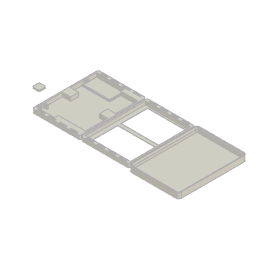
screensv16 (Autodesk Fusion 360 design; units mm, degrees)
Autodesk Fusion 360 part; units mm, degrees
sketch "Sketch1" plane through (0, 0, 0) normal (0, 0, 1) x (1, 0, 0)
  line L0 (0.0242, 17.1172) -> (73.5242, 17.1172)
  line L1 (73.5242, 17.1172) -> (73.5242, -31.8828)
  line L2 (73.5242, -31.8828) -> (0.0242, -31.8828)
  line L3 (0.0242, -31.8828) -> (0.0242, 17.1172)
  line L4 (-7.2758, 20.2172) -> (70.6242, 20.2172)
  line L5 (-7.2758, 20.2172) -> (75.7242, 20.2172)
  line L6 (75.7242, 20.2172) -> (75.7242, -34.9828)
  line L7 (-7.2758, -34.9828) -> (-7.2758, 20.2172)
  line L8 (-9.6758, 25.8172) -> (78.1242, 25.8172)
  line L9 (78.1242, 25.8172) -> (78.1242, -95.7828)
  line L10 (78.1242, -95.7828) -> (-9.6758, -95.7828)
  line L11 (-9.6758, -95.7828) -> (-9.6758, 25.8172)
  line L12 (-7.2758, -34.9828) -> (70.6242, -34.9828)
  line L13 (70.6242, -34.9828) -> (75.7242, -34.9828)
  line L14 (75.7242, -34.9828) -> (75.7242, -90.1828)
  line L15 (-7.2758, -90.1828) -> (70.6242, -90.1828)
  line L16 (70.6242, -90.1828) -> (75.7242, -90.1828)
  line L17 (-7.2758, -34.9828) -> (-7.2758, -90.1828)
  line L18 (0.0242, -38.0828) -> (73.5242, -38.0828)
  line L19 (73.5242, -38.0828) -> (73.5242, -87.0828)
  line L20 (73.5242, -87.0828) -> (0.0242, -87.0828)
  line L21 (0.0242, -87.0828) -> (0.0242, -38.0828)
  line L22 (70.9642, 22.0172) -> (57.9642, 22.0172)
  line L23 (57.9642, 22.0172) -> (57.9642, 24.0172)
  line L24 (57.9642, 24.0172) -> (70.9642, 24.0172)
  line L25 (70.9642, 24.0172) -> (70.9642, 22.0172)
  line L26 (10.4842, 22.0172) -> (-2.5158, 22.0172)
  line L27 (-2.5158, 22.0172) -> (-2.5158, 24.0172)
  line L28 (-2.5158, 24.0172) -> (10.4842, 24.0172)
  line L29 (10.4842, 24.0172) -> (10.4842, 22.0172)
  line L30 (50.8042, 22.0172) -> (37.8042, 22.0172)
  line L31 (37.8042, 22.0172) -> (37.8042, 24.0172)
  line L32 (37.8042, 24.0172) -> (50.8042, 24.0172)
  line L33 (50.8042, 24.0172) -> (50.8042, 22.0172)
  line L34 (30.6442, 22.0172) -> (17.6442, 22.0172)
  line L35 (17.6442, 22.0172) -> (17.6442, 24.0172)
  line L36 (17.6442, 24.0172) -> (30.6442, 24.0172)
  line L37 (30.6442, 24.0172) -> (30.6442, 22.0172)
  line L38 (70.9642, -93.9828) -> (57.9642, -93.9828)
  line L39 (57.9642, -93.9828) -> (57.9642, -91.9828)
  line L40 (57.9642, -91.9828) -> (70.9642, -91.9828)
  line L41 (70.9642, -91.9828) -> (70.9642, -93.9828)
  line L42 (50.8042, -93.9828) -> (37.8042, -93.9828)
  line L43 (37.8042, -93.9828) -> (37.8042, -91.9828)
  line L44 (37.8042, -91.9828) -> (50.8042, -91.9828)
  line L45 (50.8042, -91.9828) -> (50.8042, -93.9828)
  line L46 (30.6442, -93.9828) -> (17.6442, -93.9828)
  line L47 (17.6442, -93.9828) -> (17.6442, -91.9828)
  line L48 (17.6442, -91.9828) -> (30.6442, -91.9828)
  line L49 (30.6442, -91.9828) -> (30.6442, -93.9828)
  line L50 (10.4842, -93.9828) -> (-2.5158, -93.9828)
  line L51 (-2.5158, -93.9828) -> (-2.5158, -91.9828)
  line L52 (-2.5158, -91.9828) -> (10.4842, -91.9828)
  line L53 (10.4842, -91.9828) -> (10.4842, -93.9828)
  dimension "d1" = 73.5
  dimension "d2" = 49
  dimension "d7" = 3.1
  dimension "d29" = 2.4
  dimension "d40" = 3.1
  dimension "d41" = 55.2
  dimension "d44" = 5.6
  dimension "d45" = 73.5
  dimension "d46" = 49
  dimension "d47" = 3.1
  dimension "d49" = 3.1
  dimension "d52" = 87.8
  dimension "d53" = 121.6
  dimension "d56" = 55.2
  dimension "d190" = 2.4
  dimension "d191" = 2
  dimension "d192" = 2
  dimension "d193" = 5.6
  dimension "d194" = 13
  dimension "d195" = 13
  dimension "d196" = 13
  dimension "d197" = 2
  dimension "d198" = 1.8
  dimension "d199" = 7.16
  dimension "d200" = 7.16
  dimension "d201" = 7.16
  dimension "d202" = 13
  dimension "d203" = 2
  dimension "d204" = 7.16
  dimension "d205" = 13
  dimension "d206" = 13
  dimension "d207" = 13
  dimension "d208" = 13
  dimension "d209" = 2
  dimension "d210" = 2
  dimension "d211" = 2
  dimension "d212" = 2
  dimension "d213" = 7.16
  dimension "d214" = 7.16
  dimension "d215" = 7.16
  dimension "d216" = 7.16
  dimension "d217" = 1.8
  dimension "d259" = 7.3
  dimension "d260" = 2.2
  dimension "d261" = 83
  dimension "d263" = 7.3
  dimension "d264" = 87.8
  constraint horizontal L0
  constraint vertical L1
  constraint horizontal L2
  constraint vertical L3
  constraint horizontal L4
  constraint horizontal L5
  constraint vertical L6
  constraint vertical L7
  constraint horizontal L8
  constraint vertical L9
  constraint horizontal L10
  constraint perpendicular L6 L13
  constraint perpendicular L10 L14
  constraint perpendicular L14 L16
  constraint perpendicular L15 L17
  constraint perpendicular L12 L17
  constraint horizontal L18
  constraint vertical L19
  constraint horizontal L20
  constraint vertical L21
  constraint horizontal L22
  constraint vertical L23
  constraint horizontal L24
  constraint vertical L25
  constraint horizontal L26
  constraint vertical L27
  constraint horizontal L28
  constraint vertical L29
  constraint collinear L24 L28
  constraint horizontal L30
  constraint vertical L31
  constraint horizontal L32
  constraint vertical L33
  constraint collinear L24 L32
  constraint horizontal L34
  constraint vertical L35
  constraint horizontal L36
  constraint vertical L37
  constraint collinear L24 L36
  constraint horizontal L38
  constraint vertical L39
  constraint horizontal L40
  constraint vertical L41
  constraint horizontal L42
  constraint vertical L43
  constraint horizontal L44
  constraint vertical L45
  constraint horizontal L46
  constraint vertical L47
  constraint horizontal L48
  constraint vertical L49
  constraint horizontal L50
  constraint vertical L51
  constraint horizontal L52
  constraint vertical L53
  constraint collinear L38 L42
  constraint collinear L38 L46
  constraint collinear L38 L50
  measures "d1" distance of L0.start L0.end
  measures "d2" distance of L0.start L2.end
  measures "d7" distance of L0 L4
  measures "d29" distance of L6 L9
  measures "d40" distance of L2 L12
  measures "d41" distance of L4.start L7.start
  measures "d44" distance of L10 L15
  measures "d45" distance of L18.start L18.end
  measures "d46" distance of L18 L20
  measures "d47" distance of L12 L18
  measures "d49" distance of L15 L20
  measures "d52" distance of L9.end L10.end
  measures "d53" distance of L8.end L9.end
  measures "d56" distance of L7.start L15.start
  measures "d190" distance of L7 L11
  measures "d191" distance of L22.end L23.end
  measures "d192" distance of L26.start L28.end
  measures "d193" distance of L5 L8
  measures "d194" distance of L27.end L28.end
  measures "d195" distance of L23.end L24.end
  measures "d196" distance of L31.end L32.end
  measures "d197" distance of L30.end L31.end
  measures "d198" distance of L8 L24
  measures "d199" distance of L9 L25
  measures "d200" distance of L23 L33
  measures "d201" distance of L11 L27
  measures "d202" distance of L35.end L36.end
  measures "d203" distance of L34.end L35.end
  measures "d204" distance of L29 L35
  measures "d205" distance of L38.start L38.end
  measures "d206" distance of L42.start L42.end
  measures "d207" distance of L46.start L46.end
  measures "d208" distance of L50.start L50.end
  measures "d209" distance of L38.start L40.end
  measures "d210" distance of L42.start L44.end
  measures "d211" distance of L46.start L48.end
  measures "d212" distance of L50.start L52.end
  measures "d213" distance of L9 L41
  measures "d214" distance of L39 L45
  measures "d215" distance of L43 L49
  measures "d216" distance of L47 L53
  measures "d217" distance of L10 L38
  measures "d259" distance of L3 L7
  measures "d260" distance of L1 L6
  measures "d261" distance of L4.start L5.end
  measures "d263" distance of L17 L21
  measures "d264" distance of L8.start L8.end
extrude "Extrude2" add sketch "Sketch1" along normal blind 1.6 contours L4 L5 L6 L7 L12 L13 | L12 L13 L14 L15 L16 L17 | L22 L23 L24 L25 | L26 L27 L28 L29 | L30 L31 L32 L33 | L34 L35 L36 L37 | L38 L39 L40 L41 | L42 L43 L44 L45 | L46 L47 L48 L49 | L50 L51 L52 L53 makes body 1 at (-4.8425, -33.9495, 0) makes body 2 at (6.1509, 22.6838, 0) makes body 3 at (66.6309, 22.6838, 0) makes body 4 at (46.4709, 23.3505, 0) makes body 5 at (21.9775, 22.6838, 0) makes body 6 at (42.1375, -92.6495, 0) makes body 7 at (62.2975, -92.6495, 0) makes body 8 at (21.9775, -93.3162, 0) makes body 9 at (1.8175, -93.3162, 0)
extrude "Extrude4" add sketch "Sketch1" along normal blind 8 contours L8 L9 L10 L11 bodies 6 7 8 4 9 5 1 2 3
sketch "Sketch3" plane through (0, 0, 0) normal (0, 0, 1) x (1, 0, 0)
  line L0 (-7.2758, -90.1828) -> (-7.2758, 20.2172)
  line L1 (-9.6758, 25.8172) -> (-9.6758, -95.7828)
  line L2 (10.4842, 24.0172) -> (-2.5158, 24.0172)
  line L3 (-2.5158, 24.0172) -> (-2.5158, 22.0172)
  line L4 (-2.5158, 22.0172) -> (10.4842, 22.0172)
  line L5 (10.4842, 22.0172) -> (10.4842, 24.0172)
  line L6 (70.9642, 24.0172) -> (57.9642, 24.0172)
  line L7 (57.9642, 24.0172) -> (57.9642, 22.0172)
  line L8 (57.9642, 22.0172) -> (70.9642, 22.0172)
  line L9 (70.9642, 22.0172) -> (70.9642, 24.0172)
  line L10 (-7.2758, 20.2172) -> (75.7242, 20.2172)
  line L11 (78.1242, 25.8172) -> (-9.6758, 25.8172)
  line L12 (75.7242, 20.2172) -> (75.7242, -90.1828)
  line L13 (78.1242, -95.7828) -> (78.1242, 25.8172)
  line L14 (75.7242, -90.1828) -> (-7.2758, -90.1828)
  line L15 (-9.6758, -95.7828) -> (78.1242, -95.7828)
  line L16 (75.7242, -90.1828) -> (-7.2758, -90.1828)
  line L17 (-7.2758, -90.1828) -> (-7.2758, 20.2172)
  line L18 (-7.2758, 20.2172) -> (75.7242, 20.2172)
  line L19 (75.7242, 20.2172) -> (75.7242, -90.1828)
  line L20 (78.1242, -95.7828) -> (-9.105, -95.7828)
  line L21 (-9.6758, 25.8172) -> (78.1242, 25.8172)
  line L22 (78.1242, 25.8172) -> (78.1242, -95.7828)
  line L23 (70.9642, 22.0172) -> (57.9642, 22.0172)
  line L24 (57.9642, 22.0172) -> (57.9642, 24.0172)
  line L25 (57.9642, 24.0172) -> (70.9642, 24.0172)
  line L26 (70.9642, 24.0172) -> (70.9642, 22.0172)
  line L27 (10.4842, 22.0172) -> (-2.5158, 22.0172)
  line L28 (-2.5158, 22.0172) -> (-2.5158, 24.0172)
  line L29 (-2.5158, 24.0172) -> (10.4842, 24.0172)
  line L30 (10.4842, 24.0172) -> (10.4842, 22.0172)
  line L31 (26.4742, 20.2172) -> (29.4742, 20.2172)
  line L32 (38.4742, 20.2172) -> (52.2742, 20.2172)
  line L33 (75.7242, -90.1828) -> (14.7242, -90.1828)
  line L34 (5.7242, -90.1828) -> (-7.2758, -90.1828)
  line L35 (75.7242, -50.1828) -> (75.7242, -48.1828)
  line L36 (7.7242, -42.4828) -> (-7.2758, -42.4828)
  line L37 (-7.2758, -42.4828) -> (-7.2758, -27.4828)
  line L38 (-7.2758, -27.4828) -> (7.7242, -27.4828)
  line L39 (7.7242, -27.4828) -> (7.7242, -42.4828)
  line L40 (75.7242, -27.4828) -> (75.7242, -42.4828)
  line L41 (70.9642, 24.0172) -> (57.9642, 24.0172)
  line L42 (57.9642, 24.0172) -> (57.9642, 22.0172)
  line L43 (57.9642, 22.0172) -> (70.9642, 22.0172)
  line L44 (70.9642, 22.0172) -> (70.9642, 24.0172)
  line L45 (10.4842, 24.0172) -> (-2.5158, 24.0172)
  line L46 (-2.5158, 24.0172) -> (-2.5158, 22.0172)
  line L47 (-2.5158, 22.0172) -> (10.4842, 22.0172)
  line L48 (10.4842, 22.0172) -> (10.4842, 24.0172)
  line L49 (70.9642, 24.0172) -> (57.9642, 24.0172)
  line L50 (57.9642, 24.0172) -> (57.9642, 22.0172)
  line L51 (57.9642, 22.0172) -> (70.9642, 22.0172)
  line L52 (70.9642, 22.0172) -> (70.9642, 24.0172)
  line L53 (10.4842, 24.0172) -> (-2.5158, 24.0172)
  line L54 (-2.5158, 24.0172) -> (-2.5158, 22.0172)
  line L55 (-2.5158, 22.0172) -> (10.4842, 22.0172)
  line L56 (10.4842, 22.0172) -> (10.4842, 24.0172)
  line L57 (70.9642, 24.0172) -> (57.9642, 24.0172)
  line L58 (57.9642, 24.0172) -> (57.9642, 22.0172)
  line L59 (57.9642, 22.0172) -> (70.9642, 22.0172)
  line L60 (70.9642, 22.0172) -> (70.9642, 24.0172)
  line L61 (10.4842, 24.0172) -> (-2.5158, 24.0172)
  line L62 (-2.5158, 24.0172) -> (-2.5158, 22.0172)
  line L63 (-2.5158, 22.0172) -> (10.4842, 22.0172)
  line L64 (10.4842, 22.0172) -> (10.4842, 24.0172)
  line L65 (70.9642, 24.0172) -> (57.9642, 24.0172)
  line L66 (57.9642, 24.0172) -> (57.9642, 22.0172)
  line L67 (57.9642, 22.0172) -> (70.9642, 22.0172)
  line L68 (70.9642, 22.0172) -> (70.9642, 24.0172)
  line L69 (10.4842, 24.0172) -> (-2.5158, 24.0172)
  line L70 (-2.5158, 24.0172) -> (-2.5158, 22.0172)
  line L71 (-2.5158, 22.0172) -> (10.4842, 22.0172)
  line L72 (10.4842, 22.0172) -> (10.4842, 24.0172)
  line L73 (70.9642, 24.0172) -> (57.9642, 24.0172)
  line L74 (57.9642, 24.0172) -> (57.9642, 22.0172)
  line L75 (57.9642, 22.0172) -> (70.9642, 22.0172)
  line L76 (70.9642, 22.0172) -> (70.9642, 24.0172)
  line L77 (10.4842, 24.0172) -> (-2.5158, 24.0172)
  line L78 (-2.5158, 24.0172) -> (-2.5158, 22.0172)
  line L79 (-2.5158, 22.0172) -> (10.4842, 22.0172)
  line L80 (10.4842, 22.0172) -> (10.4842, 24.0172)
  line L81 (70.9642, 24.0172) -> (57.9642, 24.0172)
  line L82 (57.9642, 24.0172) -> (57.9642, 22.0172)
  line L83 (57.9642, 22.0172) -> (70.9642, 22.0172)
  line L84 (70.9642, 22.0172) -> (70.9642, 24.0172)
  line L85 (10.4842, 24.0172) -> (-2.5158, 24.0172)
  line L86 (-2.5158, 24.0172) -> (-2.5158, 22.0172)
  line L87 (-2.5158, 22.0172) -> (10.4842, 22.0172)
  line L88 (10.4842, 22.0172) -> (10.4842, 24.0172)
  line L89 (50.8042, 24.0172) -> (37.8042, 24.0172)
  line L90 (37.8042, 24.0172) -> (37.8042, 22.0172)
  line L91 (37.8042, 22.0172) -> (50.8042, 22.0172)
  line L92 (50.8042, 22.0172) -> (50.8042, 24.0172)
  line L93 (30.6442, 24.0172) -> (17.6442, 24.0172)
  line L94 (17.6442, 24.0172) -> (17.6442, 22.0172)
  line L95 (17.6442, 22.0172) -> (30.6442, 22.0172)
  line L96 (30.6442, 22.0172) -> (30.6442, 24.0172)
  line L97 (50.8042, 24.0172) -> (37.8042, 24.0172)
  line L98 (37.8042, 24.0172) -> (37.8042, 22.0172)
  line L99 (37.8042, 22.0172) -> (50.8042, 22.0172)
  line L100 (50.8042, 22.0172) -> (50.8042, 24.0172)
  line L101 (30.6442, 24.0172) -> (17.6442, 24.0172)
  line L102 (17.6442, 24.0172) -> (17.6442, 22.0172)
  line L103 (17.6442, 22.0172) -> (30.6442, 22.0172)
  line L104 (30.6442, 22.0172) -> (30.6442, 24.0172)
  line L105 (50.8042, 24.0172) -> (37.8042, 24.0172)
  line L106 (37.8042, 24.0172) -> (37.8042, 22.0172)
  line L107 (37.8042, 22.0172) -> (50.8042, 22.0172)
  line L108 (50.8042, 22.0172) -> (50.8042, 24.0172)
  line L109 (30.6442, 24.0172) -> (17.6442, 24.0172)
  line L110 (17.6442, 24.0172) -> (17.6442, 22.0172)
  line L111 (17.6442, 22.0172) -> (30.6442, 22.0172)
  line L112 (30.6442, 22.0172) -> (30.6442, 24.0172)
  line L113 (50.8042, 24.0172) -> (37.8042, 24.0172)
  line L114 (37.8042, 24.0172) -> (37.8042, 22.0172)
  line L115 (37.8042, 22.0172) -> (50.8042, 22.0172)
  line L116 (50.8042, 22.0172) -> (50.8042, 24.0172)
  line L117 (30.6442, 24.0172) -> (17.6442, 24.0172)
  line L118 (17.6442, 24.0172) -> (17.6442, 22.0172)
  line L119 (17.6442, 22.0172) -> (30.6442, 22.0172)
  line L120 (30.6442, 22.0172) -> (30.6442, 24.0172)
  line L121 (50.8042, 24.0172) -> (37.8042, 24.0172)
  line L122 (37.8042, 24.0172) -> (37.8042, 22.0172)
  line L123 (37.8042, 22.0172) -> (50.8042, 22.0172)
  line L124 (50.8042, 22.0172) -> (50.8042, 24.0172)
  line L125 (30.6442, 24.0172) -> (17.6442, 24.0172)
  line L126 (17.6442, 24.0172) -> (17.6442, 22.0172)
  line L127 (17.6442, 22.0172) -> (30.6442, 22.0172)
  line L128 (30.6442, 22.0172) -> (30.6442, 24.0172)
  line L129 (50.8042, 24.0172) -> (37.8042, 24.0172)
  line L130 (37.8042, 24.0172) -> (37.8042, 22.0172)
  line L131 (37.8042, 22.0172) -> (50.8042, 22.0172)
  line L132 (50.8042, 22.0172) -> (50.8042, 24.0172)
  line L133 (30.6442, 24.0172) -> (17.6442, 24.0172)
  line L134 (17.6442, 24.0172) -> (17.6442, 22.0172)
  line L135 (17.6442, 22.0172) -> (30.6442, 22.0172)
  line L136 (30.6442, 22.0172) -> (30.6442, 24.0172)
  line L137 (70.9642, 24.0172) -> (57.9642, 24.0172)
  line L138 (57.9642, 24.0172) -> (57.9642, 22.0172)
  line L139 (57.9642, 22.0172) -> (70.9642, 22.0172)
  line L140 (70.9642, 22.0172) -> (70.9642, 24.0172)
  line L141 (10.4842, 24.0172) -> (-2.5158, 24.0172)
  line L142 (-2.5158, 24.0172) -> (-2.5158, 22.0172)
  line L143 (-2.5158, 22.0172) -> (10.4842, 22.0172)
  line L144 (10.4842, 22.0172) -> (10.4842, 24.0172)
  line L145 (30.6442, 24.0172) -> (17.6442, 24.0172)
  line L146 (17.6442, 24.0172) -> (17.6442, 22.0172)
  line L147 (17.6442, 22.0172) -> (30.6442, 22.0172)
  line L148 (30.6442, 22.0172) -> (30.6442, 24.0172)
  line L149 (50.8042, 24.0172) -> (37.8042, 24.0172)
  line L150 (37.8042, 24.0172) -> (37.8042, 22.0172)
  line L151 (37.8042, 22.0172) -> (50.8042, 22.0172)
  line L152 (50.8042, 22.0172) -> (50.8042, 24.0172)
  line L153 (70.9642, 24.0172) -> (57.9642, 24.0172)
  line L154 (57.9642, 24.0172) -> (57.9642, 22.0172)
  line L155 (57.9642, 22.0172) -> (70.9642, 22.0172)
  line L156 (70.9642, 22.0172) -> (70.9642, 24.0172)
  line L157 (10.4842, 24.0172) -> (-2.5158, 24.0172)
  line L158 (-2.5158, 24.0172) -> (-2.5158, 22.0172)
  line L159 (-2.5158, 22.0172) -> (10.4842, 22.0172)
  line L160 (10.4842, 22.0172) -> (10.4842, 24.0172)
  line L161 (30.6442, 24.0172) -> (17.6442, 24.0172)
  line L162 (17.6442, 24.0172) -> (17.6442, 22.0172)
  line L163 (17.6442, 22.0172) -> (30.6442, 22.0172)
  line L164 (30.6442, 22.0172) -> (30.6442, 24.0172)
  line L165 (50.8042, 24.0172) -> (37.8042, 24.0172)
  line L166 (37.8042, 24.0172) -> (37.8042, 22.0172)
  line L167 (37.8042, 22.0172) -> (50.8042, 22.0172)
  line L168 (50.8042, 22.0172) -> (50.8042, 24.0172)
  line L169 (50.8042, -91.9828) -> (37.8042, -91.9828)
  line L170 (37.8042, -91.9828) -> (37.8042, -93.9828)
  line L171 (37.8042, -93.9828) -> (50.8042, -93.9828)
  line L172 (50.8042, -93.9828) -> (50.8042, -91.9828)
  line L173 (70.9642, -91.9828) -> (57.9642, -91.9828)
  line L174 (57.9642, -91.9828) -> (57.9642, -93.9828)
  line L175 (57.9642, -93.9828) -> (70.9642, -93.9828)
  line L176 (70.9642, -93.9828) -> (70.9642, -91.9828)
  line L177 (30.6442, -91.9828) -> (17.6442, -91.9828)
  line L178 (17.6442, -91.9828) -> (17.6442, -93.9828)
  line L179 (17.6442, -93.9828) -> (30.6442, -93.9828)
  line L180 (30.6442, -93.9828) -> (30.6442, -91.9828)
  line L181 (10.4842, -91.9828) -> (-2.5158, -91.9828)
  line L182 (-2.5158, -91.9828) -> (-2.5158, -93.9828)
  line L183 (-2.5158, -93.9828) -> (10.4842, -93.9828)
  line L184 (10.4842, -93.9828) -> (10.4842, -91.9828)
  line L185 (50.8042, -91.9828) -> (37.8042, -91.9828)
  line L186 (37.8042, -91.9828) -> (37.8042, -93.9828)
  line L187 (37.8042, -93.9828) -> (50.8042, -93.9828)
  line L188 (50.8042, -93.9828) -> (50.8042, -91.9828)
  line L189 (70.9642, -91.9828) -> (57.9642, -91.9828)
  line L190 (57.9642, -91.9828) -> (57.9642, -93.9828)
  line L191 (57.9642, -93.9828) -> (70.9642, -93.9828)
  line L192 (70.9642, -93.9828) -> (70.9642, -91.9828)
  line L193 (30.6442, -91.9828) -> (17.6442, -91.9828)
  line L194 (17.6442, -91.9828) -> (17.6442, -93.9828)
  line L195 (17.6442, -93.9828) -> (30.6442, -93.9828)
  line L196 (30.6442, -93.9828) -> (30.6442, -91.9828)
  line L197 (10.4842, -91.9828) -> (-2.5158, -91.9828)
  line L198 (-2.5158, -91.9828) -> (-2.5158, -93.9828)
  line L199 (-2.5158, -93.9828) -> (10.4842, -93.9828)
  line L200 (10.4842, -93.9828) -> (10.4842, -91.9828)
  line L201 (50.8042, -91.9828) -> (37.8042, -91.9828)
  line L202 (37.8042, -91.9828) -> (37.8042, -93.9828)
  line L203 (37.8042, -93.9828) -> (50.8042, -93.9828)
  line L204 (50.8042, -93.9828) -> (50.8042, -91.9828)
  line L205 (70.9642, -91.9828) -> (57.9642, -91.9828)
  line L206 (57.9642, -91.9828) -> (57.9642, -93.9828)
  line L207 (57.9642, -93.9828) -> (70.9642, -93.9828)
  line L208 (70.9642, -93.9828) -> (70.9642, -91.9828)
  line L209 (30.6442, -91.9828) -> (17.6442, -91.9828)
  line L210 (17.6442, -91.9828) -> (17.6442, -93.9828)
  line L211 (17.6442, -93.9828) -> (30.6442, -93.9828)
  line L212 (30.6442, -93.9828) -> (30.6442, -91.9828)
  line L213 (10.4842, -91.9828) -> (-2.5158, -91.9828)
  line L214 (-2.5158, -91.9828) -> (-2.5158, -93.9828)
  line L215 (-2.5158, -93.9828) -> (10.4842, -93.9828)
  line L216 (10.4842, -93.9828) -> (10.4842, -91.9828)
  line L217 (50.8042, -91.9828) -> (37.8042, -91.9828)
  line L218 (37.8042, -91.9828) -> (37.8042, -93.9828)
  line L219 (37.8042, -93.9828) -> (50.8042, -93.9828)
  line L220 (50.8042, -93.9828) -> (50.8042, -91.9828)
  line L221 (70.9642, -91.9828) -> (57.9642, -91.9828)
  line L222 (57.9642, -91.9828) -> (57.9642, -93.9828)
  line L223 (57.9642, -93.9828) -> (70.9642, -93.9828)
  line L224 (70.9642, -93.9828) -> (70.9642, -91.9828)
  line L225 (30.6442, -91.9828) -> (17.6442, -91.9828)
  line L226 (17.6442, -91.9828) -> (17.6442, -93.9828)
  line L227 (17.6442, -93.9828) -> (30.6442, -93.9828)
  line L228 (30.6442, -93.9828) -> (30.6442, -91.9828)
  line L229 (10.4842, -91.9828) -> (-2.5158, -91.9828)
  line L230 (-2.5158, -91.9828) -> (-2.5158, -93.9828)
  line L231 (-2.5158, -93.9828) -> (10.4842, -93.9828)
  line L232 (10.4842, -93.9828) -> (10.4842, -91.9828)
  line L233 (50.8042, -91.9828) -> (37.8042, -91.9828)
  line L234 (37.8042, -91.9828) -> (37.8042, -93.9828)
  line L235 (37.8042, -93.9828) -> (50.8042, -93.9828)
  line L236 (50.8042, -93.9828) -> (50.8042, -91.9828)
  line L237 (70.9642, -91.9828) -> (57.9642, -91.9828)
  line L238 (57.9642, -91.9828) -> (57.9642, -93.9828)
  line L239 (57.9642, -93.9828) -> (70.9642, -93.9828)
  line L240 (70.9642, -93.9828) -> (70.9642, -91.9828)
  line L241 (30.6442, -91.9828) -> (17.6442, -91.9828)
  line L242 (17.6442, -91.9828) -> (17.6442, -93.9828)
  line L243 (17.6442, -93.9828) -> (30.6442, -93.9828)
  line L244 (30.6442, -93.9828) -> (30.6442, -91.9828)
  line L245 (10.4842, -91.9828) -> (-2.5158, -91.9828)
  line L246 (-2.5158, -91.9828) -> (-2.5158, -93.9828)
  line L247 (-2.5158, -93.9828) -> (10.4842, -93.9828)
  line L248 (10.4842, -93.9828) -> (10.4842, -91.9828)
  line L249 (50.8042, -91.9828) -> (37.8042, -91.9828)
  line L250 (37.8042, -91.9828) -> (37.8042, -93.9828)
  line L251 (37.8042, -93.9828) -> (50.8042, -93.9828)
  line L252 (50.8042, -93.9828) -> (50.8042, -91.9828)
  line L253 (70.9642, -91.9828) -> (57.9642, -91.9828)
  line L254 (57.9642, -91.9828) -> (57.9642, -93.9828)
  line L255 (57.9642, -93.9828) -> (70.9642, -93.9828)
  line L256 (70.9642, -93.9828) -> (70.9642, -91.9828)
  line L257 (30.6442, -91.9828) -> (17.6442, -91.9828)
  line L258 (17.6442, -91.9828) -> (17.6442, -93.9828)
  line L259 (17.6442, -93.9828) -> (30.6442, -93.9828)
  line L260 (30.6442, -93.9828) -> (30.6442, -91.9828)
  line L261 (10.4842, -91.9828) -> (-2.5158, -91.9828)
  line L262 (-2.5158, -91.9828) -> (-2.5158, -93.9828)
  line L263 (-2.5158, -93.9828) -> (10.4842, -93.9828)
  line L264 (10.4842, -93.9828) -> (10.4842, -91.9828)
  line L265 (50.8042, -91.9828) -> (37.8042, -91.9828)
  line L266 (37.8042, -91.9828) -> (37.8042, -93.9828)
  line L267 (37.8042, -93.9828) -> (50.8042, -93.9828)
  line L268 (50.8042, -93.9828) -> (50.8042, -91.9828)
  line L269 (70.9642, -91.9828) -> (57.9642, -91.9828)
  line L270 (57.9642, -91.9828) -> (57.9642, -93.9828)
  line L271 (57.9642, -93.9828) -> (70.9642, -93.9828)
  line L272 (70.9642, -93.9828) -> (70.9642, -91.9828)
  line L273 (30.6442, -91.9828) -> (17.6442, -91.9828)
  line L274 (17.6442, -91.9828) -> (17.6442, -93.9828)
  line L275 (17.6442, -93.9828) -> (30.6442, -93.9828)
  line L276 (30.6442, -93.9828) -> (30.6442, -91.9828)
  line L277 (10.4842, -91.9828) -> (-2.5158, -91.9828)
  line L278 (-2.5158, -91.9828) -> (-2.5158, -93.9828)
  line L279 (-2.5158, -93.9828) -> (10.4842, -93.9828)
  line L280 (10.4842, -93.9828) -> (10.4842, -91.9828)
  line L281 (50.8042, -91.9828) -> (37.8042, -91.9828)
  line L282 (37.8042, -91.9828) -> (37.8042, -93.9828)
  line L283 (37.8042, -93.9828) -> (50.8042, -93.9828)
  line L284 (50.8042, -93.9828) -> (50.8042, -91.9828)
  line L285 (70.9642, -91.9828) -> (57.9642, -91.9828)
  line L286 (57.9642, -91.9828) -> (57.9642, -93.9828)
  line L287 (57.9642, -93.9828) -> (70.9642, -93.9828)
  line L288 (70.9642, -93.9828) -> (70.9642, -91.9828)
  line L289 (30.6442, -91.9828) -> (17.6442, -91.9828)
  line L290 (17.6442, -91.9828) -> (17.6442, -93.9828)
  line L291 (17.6442, -93.9828) -> (30.6442, -93.9828)
  line L292 (30.6442, -93.9828) -> (30.6442, -91.9828)
  line L293 (10.4842, -91.9828) -> (-2.5158, -91.9828)
  line L294 (-2.5158, -91.9828) -> (-2.5158, -93.9828)
  line L295 (-2.5158, -93.9828) -> (10.4842, -93.9828)
  line L296 (10.4842, -93.9828) -> (10.4842, -91.9828)
  line L297 (-7.2758, -77.1828) -> (-0.7758, -77.1828)
  line L298 (-0.7758, -77.1828) -> (-0.7758, -75.1828)
  line L299 (-0.7758, -75.1828) -> (-7.2758, -75.1828)
  line L300 (-7.2758, -75.1828) -> (-7.2758, -77.1828)
  line L301 (-7.2758, -5.5828) -> (42.5242, -5.5828)
  line L302 (42.5242, -5.5828) -> (42.48, 20.2172)
  line L303 (-7.2758, -2.8828) -> (-2.2758, -2.8828)
  line L304 (-2.2758, -2.8828) -> (-2.2758, 6.1172)
  line L305 (-2.2758, 6.1172) -> (-7.2758, 6.1172)
  line L306 (-7.2758, 6.1172) -> (-7.2758, -2.8828)
  line L307 (-7.2758, -7.5828) -> (44.5276, -7.5828)
  line L308 (44.5276, -7.5828) -> (44.48, 20.2206)
  line L309 (73.5242, -87.0828) -> (0.0242, -87.0828)
  line L310 (0.0242, -87.0828) -> (0.0242, -38.0828)
  line L311 (0.0242, -38.0828) -> (73.5242, -38.0828)
  line L312 (73.5242, -38.0828) -> (73.5242, -87.0828)
  line L313 (73.5242, -31.8828) -> (0.0242, -31.8828)
  line L314 (0.0242, -31.8828) -> (0.0242, 17.1172)
  line L315 (0.0242, 17.1172) -> (73.5242, 17.1172)
  line L316 (73.5242, 17.1172) -> (73.5242, -31.8828)
  line L317 (75.7242, -90.1828) -> (75.7242, 20.2172)
  line L318 (73.5242, -87.0828) -> (0.0242, -87.0828)
  line L319 (0.0242, -87.0828) -> (0.0242, -38.0828)
  line L320 (0.0242, -38.0828) -> (73.5242, -38.0828)
  line L321 (73.5242, -38.0828) -> (73.5242, -87.0828)
  line L322 (73.5242, -31.8828) -> (0.0242, -31.8828)
  line L323 (0.0242, -31.8828) -> (0.0242, 17.1172)
  line L324 (0.0242, 17.1172) -> (73.5242, 17.1172)
  line L325 (73.5242, 17.1172) -> (73.5242, -31.8828)
  line L326 (75.7242, -90.1828) -> (75.7242, 20.2172)
  line L327 (73.5242, -87.0828) -> (0.0242, -87.0828)
  line L328 (0.0242, -87.0828) -> (0.0242, -38.0828)
  line L329 (0.0242, -38.0828) -> (73.5242, -38.0828)
  line L330 (73.5242, -38.0828) -> (73.5242, -87.0828)
  line L331 (73.5242, -31.8828) -> (0.0242, -31.8828)
  line L332 (0.0242, -31.8828) -> (0.0242, 17.1172)
  line L333 (0.0242, 17.1172) -> (73.5242, 17.1172)
  line L334 (73.5242, 17.1172) -> (73.5242, -31.8828)
  line L335 (75.7242, -90.1828) -> (75.7242, 20.2172)
  line L336 (73.5242, -87.0828) -> (0.0242, -87.0828)
  line L337 (0.0242, -87.0828) -> (0.0242, -38.0828)
  line L338 (0.0242, -38.0828) -> (73.5242, -38.0828)
  line L339 (73.5242, -38.0828) -> (73.5242, -87.0828)
  line L340 (73.5242, -31.8828) -> (0.0242, -31.8828)
  line L341 (0.0242, -31.8828) -> (0.0242, 17.1172)
  line L342 (0.0242, 17.1172) -> (73.5242, 17.1172)
  line L343 (73.5242, 17.1172) -> (73.5242, -31.8828)
  line L344 (-7.2758, 20.2172) -> (-7.2758, -90.1828)
  line L345 (-7.2758, -90.1828) -> (75.7242, -90.1828)
  line L346 (75.7242, -90.1828) -> (75.7242, 20.2172)
  line L347 (75.7242, 20.2172) -> (-7.2758, 20.2172)
  line L348 (73.5242, -87.0828) -> (0.0242, -87.0828)
  line L349 (0.0242, -87.0828) -> (0.0242, -38.0828)
  line L350 (0.0242, -38.0828) -> (73.5242, -38.0828)
  line L351 (73.5242, -38.0828) -> (73.5242, -87.0828)
  line L352 (73.5242, -31.8828) -> (0.0242, -31.8828)
  line L353 (0.0242, -31.8828) -> (0.0242, 17.1172)
  line L354 (0.0242, 17.1172) -> (73.5242, 17.1172)
  line L355 (73.5242, 17.1172) -> (73.5242, -31.8828)
  line L356 (-7.2758, 20.2172) -> (-7.2758, -90.1828)
  line L357 (-7.2758, -90.1828) -> (75.7242, -90.1828)
  line L358 (75.7242, -90.1828) -> (75.7242, 20.2172)
  line L359 (75.7242, 20.2172) -> (-7.2758, 20.2172)
  line L360 (73.5242, -87.0828) -> (0.0242, -87.0828)
  line L361 (0.0242, -87.0828) -> (0.0242, -38.0828)
  line L362 (0.0242, -38.0828) -> (73.5242, -38.0828)
  line L363 (73.5242, -38.0828) -> (73.5242, -87.0828)
  line L364 (73.5242, -31.8828) -> (0.0242, -31.8828)
  line L365 (0.0242, -31.8828) -> (0.0242, 17.1172)
  line L366 (0.0242, 17.1172) -> (73.5242, 17.1172)
  line L367 (73.5242, 17.1172) -> (73.5242, -31.8828)
  line L368 (75.7242, -90.1828) -> (75.7242, 20.2172)
  line L369 (73.5242, -87.0828) -> (0.0242, -87.0828)
  line L370 (0.0242, -87.0828) -> (0.0242, -38.0828)
  line L371 (0.0242, -38.0828) -> (73.5242, -38.0828)
  line L372 (73.5242, -38.0828) -> (73.5242, -87.0828)
  line L373 (73.5242, -31.8828) -> (0.0242, -31.8828)
  line L374 (0.0242, -31.8828) -> (0.0242, 17.1172)
  line L375 (0.0242, 17.1172) -> (73.5242, 17.1172)
  line L376 (73.5242, 17.1172) -> (73.5242, -31.8828)
  line L377 (75.7242, -90.1828) -> (75.7242, 20.2172)
  line L378 (73.5242, -87.0828) -> (0.0242, -87.0828)
  line L379 (0.0242, -87.0828) -> (0.0242, -38.0828)
  line L380 (0.0242, -38.0828) -> (73.5242, -38.0828)
  line L381 (73.5242, -38.0828) -> (73.5242, -87.0828)
  line L382 (73.5242, -31.8828) -> (0.0242, -31.8828)
  line L383 (0.0242, -31.8828) -> (0.0242, 17.1172)
  line L384 (0.0242, 17.1172) -> (73.5242, 17.1172)
  line L385 (73.5242, 17.1172) -> (73.5242, -31.8828)
  line L386 (-7.2758, 20.2172) -> (-7.2758, -90.1828)
  line L387 (-7.2758, -90.1828) -> (75.7242, -90.1828)
  line L388 (75.7242, -90.1828) -> (75.7242, 20.2172)
  line L389 (75.7242, 20.2172) -> (-7.2758, 20.2172)
  line L390 (75.7242, 20.2172) -> (44.492, 20.2172)
  line L391 (44.492, 20.2172) -> (44.492, 13.2172)
  line L392 (44.492, 13.2172) -> (75.7242, 13.2172)
  line L393 (75.7242, 13.2172) -> (75.7242, 20.2172)
  line L394 (75.7242, -90.1828) -> (25.7242, -90.1828)
  line L395 (25.7242, -90.1828) -> (25.7242, -83.1828)
  line L396 (25.7242, -83.1828) -> (75.7242, -83.1828)
  line L397 (75.7242, -83.1828) -> (75.7242, -90.1828)
  line L398 (75.7242, -42.4828) -> (60.7242, -42.4828)
  line L399 (75.7242, -27.4828) -> (60.7242, -27.4828)
  line L400 (60.7242, -27.4828) -> (60.7242, -42.4828)
  line L401 (-7.2758, -34.9828) -> (-7.2758, 20.2172)
  line L402 (-7.2758, 20.2172) -> (70.6242, 20.2172)
  dimension "d172" = 15
  dimension "d173" = 15
  dimension "d175" = 15
  dimension "d222" = 6.5
  dimension "d223" = 2
  dimension "d224" = 13
  dimension "d238" = 25.8
  dimension "d239" = 5
  dimension "d240" = 9
  dimension "d241" = 2.7
  dimension "d242" = 49.8
  dimension "d243" = 2
  dimension "d266" = 7
  dimension "d267" = 7
  dimension "d268" = 15
  dimension "d270" = 50
  constraint horizontal L16
  constraint vertical L17
  constraint horizontal L18
  constraint vertical L19
  constraint coincident L0.end L10.start
  constraint coincident L12.end L14.start
  constraint horizontal L20
  constraint horizontal L21
  constraint vertical L22
  constraint coincident L1.start L11.end
  constraint coincident L13.start L15.end
  constraint horizontal L23
  constraint vertical L24
  constraint horizontal L25
  constraint vertical L26
  constraint coincident L6.end L7.start
  constraint coincident L8.end L9.start
  constraint horizontal L27
  constraint vertical L28
  constraint horizontal L29
  constraint vertical L30
  constraint coincident L2.end L3.start
  constraint coincident L4.end L5.start
  constraint horizontal L33
  constraint horizontal L34
  constraint coincident L0.start L14.end
  constraint vertical L35
  constraint collinear L19 L35
  constraint horizontal L36
  constraint vertical L37
  constraint horizontal L38
  constraint vertical L39
  constraint midpoint L17 L37
  constraint vertical L40
  constraint midpoint L19 L40
  constraint horizontal L297
  constraint vertical L298
  constraint horizontal L299
  constraint vertical L300
  constraint horizontal L303
  constraint vertical L304
  constraint horizontal L305
  constraint vertical L306
  constraint coincident L17 L303.start
  constraint horizontal L390
  constraint vertical L391
  constraint horizontal L392
  constraint vertical L393
  constraint coincident L308 L391.end
  constraint coincident L10.end L12.start
  constraint horizontal L394
  constraint vertical L395
  constraint horizontal L396
  constraint vertical L397
  constraint horizontal L398
  constraint horizontal L399
  constraint perpendicular L398 L400
  constraint coincident L301.start L401
  constraint coincident L302.end L402
  measures "d172" distance of L36.start L36.end
  measures "d173" distance of L36.start L38.end
  measures "d175" distance of L40.end L40.start
  measures "d222" distance of L297.start L297.end
  measures "d223" distance of L297.start L299.end
  measures "d224" distance of L0.start L297.start
  measures "d238" distance of L301.end L302.end
  measures "d239" distance of L303.start L303.end
  measures "d240" distance of L303.start L305.end
  measures "d241" distance of L301 L303
  measures "d242" distance of L301.start L301.end
  measures "d266" distance of L10.end L392.end
  measures "d267" distance of L12.end L396.end
  measures "d268" distance of L40.end L398.end
  measures "d270" distance of L395.end L396.end
extrude "Extrude7" add sketch "Sketch3" along normal blind 1 separate body contours L0 L14 L16 L17 L33 L34 L36 L297 L298 L299 L309 L310 L318 L319 L327 L328 L336 L337 L344 L345 L348 L349 L356 L357 L360 L361 L369 L370 L378 L379 L386 L387 L395 | L0 L17 L297 L298 L299 L300 L344 L356 L386 | L0 L17 L36 L37 L38 L39 L310 L311 L313 L314 L319 L320 L322 L323 L328 L329 L331 L332 L337 L338 L340 L341 L344 L349 L350 L352 L353 L356 L361 L362 L364 L365 L370 L371 L373 L374 L379 L380 L382 L383 L386 L401 | L12 L14 L16 L19 L33 L309 L312 L317 L318 L321 L326 L327 L330 L335 L336 L339 L345 L346 L348 L351 L357 L358 L360 L363 L368 L369 L372 L377 L378 L381 L387 L388 L394 L395 L396 L397 | L36 L39 L310 L311 L319 L320 L328 L329 L337 L338 L349 L350 L361 L362 L370 L371 L379 L380 | L36 L39 L309 L310 L311 L312 L318 L319 L320 L321 L327 L328 L329 L330 L336 L337 L338 L339 L348 L349 L350 L351 L360 L361 L362 L363 L369 L370 L371 L372 L378 L379 L380 L381 L395 L396 L398 L400 | L309 L312 L318 L321 L327 L330 L336 L339 L348 L351 L360 L363 L369 L372 L378 L381 L395 L396 | L0 L17 L38 L307 L314 L323 L332 L341 L344 L353 L356 L365 L374 L383 L386 L401 | L12 L19 L35 L312 L317 L321 L326 L330 L335 L339 L346 L351 L358 L363 L368 L372 L377 L381 L388 L396 L398 | L0 L17 L301 L307 L314 L323 L332 L341 L344 L353 L356 L365 L374 L383 L386 L401 | L38 L39 L307 L308 L313 L314 L316 L322 L323 L325 L331 L332 L334 L340 L341 L343 L352 L353 L355 L364 L365 L367 L373 L374 L376 L382 L383 L385 L392 L399 L400 | L38 L39 L313 L314 L322 L323 L331 L332 L340 L341 L352 L353 L364 L365 L373 L374 L382 L383 | L39 L311 L313 L320 L322 L329 L331 L338 L340 L350 L352 L362 L364 L371 L373 L380 L382 L400 | L0 L10 L17 L18 L31 L32 L301 L302 L303 L304 L305 L314 L315 L323 L324 L332 L333 L341 L342 L344 L347 L353 L354 L356 L359 L365 L366 L374 L375 L383 L384 L386 L389 L401 L402 | L301 L302 L307 L308 L314 L315 L323 L324 L332 L333 L341 L342 L353 L354 L365 L366 L374 L375 L383 L384 | L12 L19 L40 L311 L312 L313 L316 L317 L320 L321 L322 L325 L326 L329 L330 L331 L334 L335 L338 L339 L340 L343 L346 L350 L351 L352 L355 L358 L362 L363 L364 L367 L368 L371 L372 L373 L376 L377 L380 L381 L382 L385 L388 L398 L399 L400 | L311 L312 L320 L321 L329 L330 L338 L339 L350 L351 L362 L363 L371 L372 L380 L381 L398 L400 | L0 L17 L303 L304 L305 L306 L344 L356 L386 L401 | L301 L302 L314 L315 L323 L324 L332 L333 L341 L342 L353 L354 L365 L366 L374 L375 L383 L384 | L313 L316 L322 L325 L331 L334 L340 L343 L352 L355 L364 L367 L373 L376 L382 L385 L399 L400 | L308 L315 L324 L333 L342 L354 L366 L375 L384 L391 | L315 L316 L324 L325 L333 L334 L342 L343 L354 L355 L366 L367 L375 L376 L384 L385 L391 L392 | L12 L19 L316 L317 L325 L326 L334 L335 L343 L346 L355 L358 L367 L368 L376 L377 L385 L388 L392 L399 | L10 L18 L32 L302 L308 L315 L324 L333 L342 L347 L354 L359 L366 L375 L384 L389 L402 | L10 L18 L32 L308 L315 L324 L333 L342 L347 L354 L359 L366 L375 L384 L389 L391 L402 | L10 L12 L18 L19 L32 L315 L316 L317 L324 L325 L326 L333 L334 L335 L342 L343 L346 L347 L354 L355 L358 L359 L366 L367 L368 L375 L376 L377 L384 L385 L388 L389 L390 L391 L392 L393 L402 | L1 L11 L13 L15 L20 L21 L22 | L2 L3 L4 L5 L27 L28 L29 L30 L45 L46 L47 L48 L53 L54 L55 L56 L61 L62 L63 L64 L69 L70 L71 L72 L77 L78 L79 L80 L85 L86 L87 L88 L141 L142 L143 L144 L157 L158 L159 L160 | L6 L7 L8 L9 L23 L24 L25 L26 L41 L42 L43 L44 L49 L50 L51 L52 L57 L58 L59 L60 L65 L66 L67 L68 L73 L74 L75 L76 L81 L82 L83 L84 L137 L138 L139 L140 L153 L154 L155 L156 | L89 L90 L91 L92 L97 L98 L99 L100 L105 L106 L107 L108 L113 L114 L115 L116 L121 L122 L123 L124 L129 L130 L131 L132 L149 L150 L151 L152 L165 L166 L167 L168 | L93 L94 L95 L96 L101 L102 L103 L104 L109 L110 L111 L112 L117 L118 L119 L120 L125 L126 L127 L128 L133 L134 L135 L136 L145 L146 L147 L148 L161 L162 L163 L164 | L169 L170 L171 L172 L185 L186 L187 L188 L201 L202 L203 L204 L217 L218 L219 L220 L233 L234 L235 L236 L249 L250 L251 L252 L265 L266 L267 L268 L281 L282 L283 L284 | L173 L174 L175 L176 L189 L190 L191 L192 L205 L206 L207 L208 L221 L222 L223 L224 L237 L238 L239 L240 L253 L254 L255 L256 L269 L270 L271 L272 L285 L286 L287 L288 | L177 L178 L179 L180 L193 L194 L195 L196 L209 L210 L211 L212 L225 L226 L227 L228 L241 L242 L243 L244 L257 L258 L259 L260 L273 L274 L275 L276 L289 L290 L291 L292 | L181 L182 L183 L184 L197 L198 L199 L200 L213 L214 L215 L216 L229 L230 L231 L232 L245 L246 L247 L248 L261 L262 L263 L264 L277 L278 L279 L280 L293 L294 L295 L296 makes body 10
extrude "Extrude8" add sketch "Sketch3" along normal blind 2.6 contours L0 L17 L301 L307 L314 L323 L332 L341 L344 L353 L356 L365 L374 L383 L386 L401 | L301 L302 L307 L308 L314 L315 L323 L324 L332 L333 L341 L342 L353 L354 L365 L366 L374 L375 L383 L384 | L10 L18 L32 L302 L308 L315 L324 L333 L342 L347 L354 L359 L366 L375 L384 L389 L402 bodies 10
extrude "Extrude9" add sketch "Sketch3" along normal blind 8 contours L0 L17 L297 L298 L299 L300 L344 L356 L386 | L0 L17 L36 L37 L38 L39 L310 L311 L313 L314 L319 L320 L322 L323 L328 L329 L331 L332 L337 L338 L340 L341 L344 L349 L350 L352 L353 L356 L361 L362 L364 L365 L370 L371 L373 L374 L379 L380 L382 L383 L386 L401 | L12 L14 L16 L19 L33 L309 L312 L317 L318 L321 L326 L327 L330 L335 L336 L339 L345 L346 L348 L351 L357 L358 L360 L363 L368 L369 L372 L377 L378 L381 L387 L388 L394 L395 L396 L397 | L36 L39 L310 L311 L319 L320 L328 L329 L337 L338 L349 L350 L361 L362 L370 L371 L379 L380 | L309 L312 L318 L321 L327 L330 L336 L339 L348 L351 L360 L363 L369 L372 L378 L381 L395 L396 | L38 L39 L313 L314 L322 L323 L331 L332 L340 L341 L352 L353 L364 L365 L373 L374 L382 L383 | L12 L19 L40 L311 L312 L313 L316 L317 L320 L321 L322 L325 L326 L329 L330 L331 L334 L335 L338 L339 L340 L343 L346 L350 L351 L352 L355 L358 L362 L363 L364 L367 L368 L371 L372 L373 L376 L377 L380 L381 L382 L385 L388 L398 L399 L400 | L311 L312 L320 L321 L329 L330 L338 L339 L350 L351 L362 L363 L371 L372 L380 L381 L398 L400 | L313 L316 L322 L325 L331 L334 L340 L343 L352 L355 L364 L367 L373 L376 L382 L385 L399 L400 | L315 L316 L324 L325 L333 L334 L342 L343 L354 L355 L366 L367 L375 L376 L384 L385 L391 L392 | L10 L12 L18 L19 L32 L315 L316 L317 L324 L325 L326 L333 L334 L335 L342 L343 L346 L347 L354 L355 L358 L359 L366 L367 L368 L375 L376 L377 L384 L385 L388 L389 L390 L391 L392 L393 L402 | L1 L11 L13 L15 L20 L21 L22 bodies 10
move_body "Move1" bodies 10 to x (1, 0, 0) y (0, 1, 0) z (0, 0, 1) at (-90, 0, 0)
sketch "Sketch6" plane through (-99.6758, 0, 0) normal (-1, 0, 0) x (0, -1, 0)
  line L0 (-25.8172, 0) -> (95.7828, 0)
  line L1 (95.7828, 0) -> (95.7828, 8)
  line L2 (95.7828, 8) -> (-25.8172, 8)
  line L3 (-25.8172, 8) -> (-25.8172, 0)
  line L4 (80.3828, 7) -> (86.9828, 7)
  line L5 (86.9828, 7) -> (86.9828, 2.3)
  line L6 (86.9828, 2.3) -> (80.3828, 2.3)
  line L7 (80.3828, 2.3) -> (80.3828, 7)
  line L8 (90.1828, 1) -> (90.1828, 8)
  line L9 (77.1828, 1) -> (77.1828, 8)
  line L10 (77.1828, 1) -> (90.1828, 1)
  line L11 (2.8828, 0) -> (2.8828, 8.0001) construction
  line L12 (-6.1172, 0) -> (-6.1172, 8.3009) construction
  line L13 (-6.1172, 5.8) -> (2.8828, 5.8)
  line L14 (2.8828, 5.8) -> (2.8828, 2.3)
  line L15 (2.8828, 2.3) -> (-6.1172, 2.3)
  line L16 (-6.1172, 2.3) -> (-6.1172, 5.8)
  line L17 (-20.2172, 1) -> (5.5828, 1)
  line L18 (-6.1172, 0) -> (2.8828, 0)
  dimension "d227" = 3.2
  dimension "d228" = 3.2
  dimension "d229" = 1.3
  dimension "d230" = 1
  dimension "d246" = 1.3
  dimension "d247" = 3.5
  constraint horizontal L4
  constraint vertical L5
  constraint horizontal L6
  constraint vertical L7
  constraint vertical L11
  constraint vertical L12
  constraint horizontal L13
  constraint vertical L14
  constraint horizontal L15
  constraint vertical L16
  constraint coincident L12.start L18.start
  constraint coincident L11.start L18.end
  constraint collinear L12 L16
  constraint collinear L11 L14
  measures "d227" distance of L5 L8
  measures "d228" distance of L7 L9
  measures "d229" distance of L6 L10
  measures "d230" distance of L2 L4
  measures "d246" distance of L15 L17
  measures "d247" distance of L13.end L14.end
extrude "Extrude13" cut sketch "Sketch6" against normal up to surface (2.4 mm away) contours L4 L5 L6 L7 | L13 L14 L15 L16 bodies 10
chamfer "Chamfer3" distance 1.2 angle 45 8 edges at (36.7742, -38.0828, 0) (73.5242, -62.5828, 0) (73.5242, -7.3828, 0) (36.7742, -31.8828, 0) (36.7742, 17.1172, 0) (0.0242, -7.3828, 0) (0.0242, -62.5828, 0) (36.7742, -87.0828, 0) on bodies 6
fillet "Fillet3" radius 3 8 edges at (-11.8758, 25.8172, 4) (-99.6758, 25.8172, 4) (-99.6758, -95.7828, 4) (-11.8758, -95.7828, 4) (-9.6758, -95.7828, 4) (78.1242, -95.7828, 4) (78.1242, 25.8172, 4) (-9.6758, 25.8172, 4) on bodies 6 10
fillet "Fillet3" radius 1.4 8 edges at (-99.6758, -34.9828, 0) (-55.7758, 25.8172, 0) (-55.7758, -95.7828, 0) (-11.8758, -34.9828, 0) (-9.6758, -34.9828, 0) (34.2242, -95.7828, 0) (78.1242, -34.9828, 0) (34.2242, 25.8172, 0) on bodies 6 10
fillet "Fillet3" radius 1.5 4 edges at (-98.4758, 6.1172, 5.8) (-98.4758, 6.1172, 2.3) (-98.4758, -2.8828, 2.3) (-98.4758, -2.8828, 5.8) on bodies 6 10
sketch "Sketch4" plane through (0, 0, 0) normal (0, 0, 1) x (1, 0, 0)
  line L0 (-127.429, -55.23) -> (-140.229, -55.23)
  line L1 (-140.229, -55.23) -> (-140.229, -42.43)
  line L2 (-140.229, -42.43) -> (-127.429, -42.43)
  line L3 (-127.429, -42.43) -> (-127.429, -55.23)
  dimension "d184" = 12.8
  dimension "d185" = 12.8
  constraint horizontal L0
  constraint vertical L1
  constraint horizontal L2
  constraint vertical L3
  measures "d184" distance of L0.start L0.end
  measures "d185" distance of L0.start L2.end
extrude "Extrude11" add sketch "Sketch4" along normal blind 2 separate body makes body 11
fillet "Fillet1" radius 2 4 edges at (-140.229, -42.43, 1) (-140.229, -55.23, 1) (-127.429, -42.43, 1) (-127.429, -55.23, 1) on bodies 11
sketch "Sketch8" plane through (0, 0, 0) normal (0, 0, 1) x (1, 0, 0)
  line L0 (-2.5158, -91.9828) -> (10.4842, -91.9828)
  line L1 (10.4842, -91.9828) -> (10.4842, -93.9828)
  line L2 (10.4842, -93.9828) -> (-2.5158, -93.9828)
  line L3 (-2.5158, -93.9828) -> (-2.5158, -91.9828)
  line L4 (17.6442, -91.9828) -> (30.6442, -91.9828)
  line L5 (30.6442, -91.9828) -> (30.6442, -93.9828)
  line L6 (30.6442, -93.9828) -> (17.6442, -93.9828)
  line L7 (17.6442, -93.9828) -> (17.6442, -91.9828)
  line L8 (37.8042, -91.9828) -> (50.8042, -91.9828)
  line L9 (50.8042, -91.9828) -> (50.8042, -93.9828)
  line L10 (50.8042, -93.9828) -> (37.8042, -93.9828)
  line L11 (37.8042, -93.9828) -> (37.8042, -91.9828)
  line L12 (57.9642, -91.9828) -> (70.9642, -91.9828)
  line L13 (70.9642, -91.9828) -> (70.9642, -93.9828)
  line L14 (70.9642, -93.9828) -> (57.9642, -93.9828)
  line L15 (57.9642, -93.9828) -> (57.9642, -91.9828)
  line L16 (17.6442, 24.0172) -> (30.6442, 24.0172)
  line L17 (30.6442, 24.0172) -> (30.6442, 22.0172)
  line L18 (30.6442, 22.0172) -> (17.6442, 22.0172)
  line L19 (17.6442, 22.0172) -> (17.6442, 24.0172)
  line L20 (37.8042, 24.0172) -> (50.8042, 24.0172)
  line L21 (50.8042, 24.0172) -> (50.8042, 22.0172)
  line L22 (50.8042, 22.0172) -> (37.8042, 22.0172)
  line L23 (37.8042, 22.0172) -> (37.8042, 24.0172)
  line L24 (57.9642, 24.0172) -> (70.9642, 24.0172)
  line L25 (70.9642, 24.0172) -> (70.9642, 22.0172)
  line L26 (70.9642, 22.0172) -> (57.9642, 22.0172)
  line L27 (57.9642, 22.0172) -> (57.9642, 24.0172)
  line L28 (-2.5158, 24.0172) -> (10.4842, 24.0172)
  line L29 (10.4842, 24.0172) -> (10.4842, 22.0172)
  line L30 (10.4842, 22.0172) -> (-2.5158, 22.0172)
  line L31 (-2.5158, 22.0172) -> (-2.5158, 24.0172)
  line L32 (-7.2758, -90.1828) -> (-7.2758, 20.2172)
  line L33 (-7.2758, 20.2172) -> (75.7242, 20.2172)
  line L34 (75.7242, 20.2172) -> (75.7242, -90.1828)
  line L35 (75.7242, -90.1828) -> (-7.2758, -90.1828)
  arc A0 (-9.6758, -92.7828) -> (-6.6758, -95.7828) centre (-6.6758, -92.7828) ccw
  line L36 (-6.6758, -95.7828) -> (75.1242, -95.7828)
  arc A1 (75.1242, -95.7828) -> (78.1242, -92.7828) centre (75.1242, -92.7828) ccw
  line L37 (78.1242, -92.7828) -> (78.1242, 22.8172)
  arc A2 (78.1242, 22.8172) -> (75.1242, 25.8172) centre (75.1242, 22.8172) ccw
  line L38 (75.1242, 25.8172) -> (-6.6758, 25.8172)
  arc A3 (-6.6758, 25.8172) -> (-9.6758, 22.8172) centre (-6.6758, 22.8172) ccw
  line L39 (-9.6758, 22.8172) -> (-9.6758, -92.7828)
  line L40 (-6.6758, -97.7828) -> (75.1242, -97.7828)
  arc A4 (75.1242, -97.7828) -> (80.1242, -92.7828) centre (75.1242, -92.7828) ccw
  line L41 (80.1242, -92.7828) -> (80.1242, 22.8172)
  arc A5 (80.1242, 22.8172) -> (75.1242, 27.8172) centre (75.1242, 22.8172) ccw
  line L42 (75.1242, 27.8172) -> (-6.6758, 27.8172)
  arc A6 (-6.6758, 27.8172) -> (-11.6758, 22.8172) centre (-6.6758, 22.8172) ccw
  line L43 (-11.6758, 22.8172) -> (-11.6758, -92.7828)
  arc A7 (-11.6758, -92.7828) -> (-6.6758, -97.7828) centre (-6.6758, -92.7828) ccw
  line L44 (-6.6758, -95.8828) -> (75.1242, -95.8828)
  arc A8 (75.1242, -95.8828) -> (78.2242, -92.7828) centre (75.1242, -92.7828) ccw
  line L45 (78.2242, -92.7828) -> (78.2242, 22.8172)
  arc A9 (78.2242, 22.8172) -> (75.1242, 25.9172) centre (75.1242, 22.8172) ccw
  line L46 (75.1242, 25.9172) -> (-6.6758, 25.9172)
  arc A10 (-6.6758, 25.9172) -> (-9.7758, 22.8172) centre (-6.6758, 22.8172) ccw
  line L47 (-9.7758, 22.8172) -> (-9.7758, -92.7828)
  arc A11 (-9.7758, -92.7828) -> (-6.6758, -95.8828) centre (-6.6758, -92.7828) ccw
  dimension "d278" = 2
  dimension "d285" = 0.1
extrude "Extrude14" add sketch "Sketch8" against normal blind 1.2 separate body contours L0 L1 L2 L3 | L4 L5 L6 L7 | L8 L9 L10 L11 | L12 L13 L14 L15 | L16 L17 L18 L19 | L20 L21 L22 L23 | L24 L25 L26 L27 | L28 L29 L30 L31 | L32 L33 L34 L35 | A0 L36 A1 L37 A2 L38 A3 L39 | L40 A4 L41 A5 L42 A6 L43 A7 | L44 A8 L45 A9 L46 A10 L47 A11 makes body 12
extrude "Extrude15" add sketch "Sketch8" along normal blind 9 contours L40 A4 L41 A5 L42 A6 L43 A7 bodies 12
chamfer "Chamfer4" distance 0.8 distance2 4 8 edges at (78.2242, -34.9828, 9) (77.3162, -94.9749, 9) (34.2242, -95.8828, 9) (-8.8678, -94.9749, 9) (-9.7758, -34.9828, 9) (-8.8678, 25.0092, 9) (34.2242, 25.9172, 9) (77.3162, 25.0092, 9) measured on face at (-11.0425, -15.7162, 9) measured on face at (-11.0425, -15.7162, 9) measured on face at (-11.0425, -15.7162, 9) measured on face at (-11.0425, -15.7162, 9) measured on face at (-11.0425, -15.7162, 9) measured on face at (-11.0425, -15.7162, 9) measured on face at (-11.0425, -15.7162, 9) measured on face at (-11.0425, -15.7162, 9) on bodies 12
move_body "Move2" bodies 12 to x (1, 0, 0) y (0, 1, 0) z (0, 0, 1) at (92, 0, 0)
equation "d26 = 4.8 mm"
equation "d40 = d7"
equation "d44 = d193"
equation "d45 = d1"
equation "d46 = d2"
equation "d47 = d7"
equation "d49 = d7"
equation "d63 = 1.2 mm"
equation "d85 = ( d26 - d63 ) / 2"
equation "d86 = 90.00 mm"
equation "d87 = ( d53 - d86 ) / 2"
equation "d190 = d29"
equation "d191 = d192"
equation "d195 = d194"
equation "d196 = d194"
equation "d197 = d192"
equation "d198 = ( d193 - d192 ) / 2"
equation "d199 = d213"
equation "d200 = d199"
equation "d201 = d199"
equation "d202 = d194"
equation "d203 = d192"
equation "d204 = d199"
equation "d205 = d194"
equation "d206 = d194"
equation "d207 = d194"
equation "d208 = d194"
equation "d209 = d192"
equation "d210 = d192"
equation "d211 = d192"
equation "d212 = d192"
equation "d213 = ( d52 - ( d205 * 4 ) ) / 5"
equation "d214 = d213"
equation "d215 = d213"
equation "d216 = d213"
equation "d217 = d198"
equation "d228 = d227"
equation "d263 = d259"
